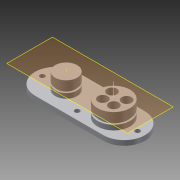
# Autodesk Inventor part: Connector
Saved by Autodesk Inventor 2014 SP2 (Build 180246200, 246)
## iProperties
Created: 2015-09-17
Part Number: Connector
Material: ABS Plastic
Document SubType Name: Modeling
Designer: Lukasz Szmit
Density: 1.06 g/cm^3
Appearance: Smooth - White
Author: Lukasz Szmit
Autodesk Inventor part; units mm, degrees
ref_plane "YZ Plane" through (0, 0, 0) normal (1, 0, 0) x (0, 1, 0)
ref_plane "XZ Plane" through (0, 0, 0) normal (0, 1, 0) x (-1, 0, 0)
sketch "Slot" plane through (0, 0, 0) normal (0, 0, 1) x (1, 0, 0)
  line L0 (-28, 17) -> (28, 17)
  line L1 (45, 0) -> (45, 0)
  line L2 (28, -17) -> (-28, -17)
  line L3 (-45, 0) -> (-45, 0)
  arc A0 (-28, 17) -> (-28, -17) centre (-28, 0) ccw
  arc A1 (28, -17) -> (28, 17) centre (28, 0) ccw
  point P0 (0, 0)
  point P1 (-45, 17)
  point P2 (45, 17)
  point P3 (-45, -17)
  dimension "d0" = 90
  dimension "d1" = 34
  dimension "d2" = 17
  dimension "d4" = 17
  dimension "d6" = 90
  dimension "d19" = 56
  dimension "d20" = 28
  constraints: 8 end point, 8 point on circle, 6 point on line, 4 tangent, 2 centre point, 2 perpendicular
  measures "d0" distance of point (-45, 17) point (45, 17)
  measures "d1" distance of point (-45, -17) point (-45, 17)
  measures "d2" distance from line of point (0, 0) L0
  measures "d4" radius of A0
  measures "d6" horizontal distance of point (45, 17) point (-45, -17)
  measures "d19" distance of A1.centre A0.centre
  measures "d20" distance of point (0, 0) A0.centre
sketch "Holes" plane through (0, 0, 0) normal (0, 0, 1) x (1, 0, 0)
  circle A0 centre (-39, 0) radius 2
  circle A1 centre (39, 0) radius 2
  circle A2 centre (0, -10.5) radius 2
  circle A3 centre (0, 10.5) radius 2
  point P0 (0, 0)
  point P1 (-3.3578, 23.5)
  dimension "d7" = 4
  dimension "d8" = 4
  dimension "d9" = 4
  dimension "d10" = 4
  dimension "d11" = 78
  dimension "d16" = 21
  dimension "d17" = 39
  constraints: 4 centre point
  measures "d7" diameter of A0
  measures "d8" diameter of A2
  measures "d9" diameter of A1
  measures "d10" diameter of A3
  measures "d11" distance of A1.centre A0.centre
  measures "d16" distance of A3.centre A2.centre
  measures "d17" horizontal distance of A1.centre A2.centre
extrude "Extrusion1" add sketch "Slot" against normal blind 4
hole "Hole1" at (0, 10.5, 0) at (39, 0, 0) at (0, -10.5, 0) at (-39, 0, 0) direction (0, 0, -1) diameter 4 end through all
ref_plane "Work Plane1" through (0, 0, 13) normal (0, 0, 1) x (1, 0, 0)
sketch "Socket Outline" plane through (0, 0, 13) normal (0, 0, 1) x (1, 0, 0)
  line L0 (-19.5, 12) -> (19.5, 12) construction
  line L1 (31.5, 0) -> (31.5, 0) construction
  line L2 (19.5, -12) -> (-19.5, -12) construction
  line L3 (-31.5, 0) -> (-31.5, 0) construction
  arc A0 (-19.5, 12) -> (-19.5, -12) centre (-19.5, 0) ccw construction
  arc A1 (19.5, -12) -> (19.5, 12) centre (19.5, 0) ccw construction
  point P0 (0, 0)
  point P1 (-31.5, 12)
  point P2 (31.5, 12)
  point P3 (-31.5, -12)
  dimension "d31" = 63
  dimension "d32" = 24
  dimension "d33" = 12
  dimension "d34" = 12
  dimension "d35" = 63
  dimension "d36" = 39
  dimension "d37" = 19.5
  constraints: 8 end point, 8 point on circle, 6 point on line, 4 tangent, 2 centre point, 2 perpendicular, 1 parallel
  measures "d31" distance of point (-31.5, 12) point (31.5, 12)
  measures "d32" distance of point (-31.5, -12) point (-31.5, 12)
  measures "d33" distance from line of point (0, 0) L0
  measures "d34" radius of A0
  measures "d35" horizontal distance of point (31.5, 12) point (-31.5, -12)
  measures "d36" distance of A1.centre A0.centre
  measures "d37" distance of point (0, 0) A0.centre
sketch "Small Socket" plane through (0, 0, 13) normal (0, 0, 1) x (1, 0, 0)
  circle A0 centre (-19.5, 0) radius 0.0027
  circle A1 centre (-19.5, 0) radius 9
  circle A2 centre (-39, 0) radius 2 projected
  point P0 (0, 0)
  dimension "d38" = 18
  dimension "d40" = 19.5
  dimension "d43" = 19.5
  constraints: 2 centre point, 1 coincident
  measures "d38" diameter of A1
  measures "d40" distance of A1.centre A2.centre
  measures "d43" distance of point (0, 0) A0.centre
sketch "Big Socket" plane through (0, 0, 13) normal (0, 0, 1) x (1, 0, 0)
  circle A0 centre (19.5, 0) radius 13.25
  circle A1 centre (39, 0) radius 2 projected
  point P0 (0, 0)
  dimension "d39" = 26.5
  dimension "d41" = 19.5
  dimension "d42" = 19.5
  constraints: 1 centre point
  measures "d39" diameter of A0
  measures "d41" distance of A1.centre A0.centre
  measures "d42" distance of point (0, 0) A0.centre
extrude "Extrusion2" add sketch "Small Socket" against normal blind 13 contours A1
extrude "Extrusion3" add sketch "Big Socket" against normal blind 13 contours A0
ref_plane "Work Plane3" through (-19.5, 0, 13) normal (1, 0, 0) x (0, 1, 0)
sketch "Sketch7" plane through (-19.5, 0, 13) normal (1, 0, 0) x (0, 1, 0)
  line L0 (-9, -13) -> (-9, 0) construction
  line L1 (-9, 0) -> (-0.0027, 0) construction
  line L2 (-0.0027, 0) -> (-0.0027, -13) construction
  line L3 (-0.0027, -13) -> (0.0027, -13) construction
  line L4 (0.0027, -13) -> (0.0027, 0) construction
  line L5 (0.0027, 0) -> (9, 0) construction
  line L6 (9, 0) -> (9, -13) construction
  line L7 (9, -13) -> (17, -13) construction
  line L8 (17, -13) -> (17, -17) construction
  line L9 (17, -17) -> (-17, -17) construction
  line L10 (-17, -17) -> (-17, -13) construction
  line L11 (-17, -13) -> (-9, -13) construction
  line L12 (9, -7.2) -> (7.5, -7.2)
  line L13 (7.5, -7.2) -> (7.5, -9)
  line L14 (7.5, -9) -> (9, -9)
  line L15 (9, -9) -> (9, -7.2)
  line L16 (0, 3.4) -> (0, -20.4) projected
  point P0 (0, -13)
  dimension "d53" = 1.5
  dimension "d54" = 1.8
  dimension "d55" = 4
  constraints: 8 end point, 1 perpendicular, 1 point on line
  measures "d53" distance of L12.start L12.end
  measures "d54" distance of L12.end L13.end
  measures "d55" distance between parallel lines of L7 L14
revolve "Revolution2" cut sketch "Sketch7" angle 360 about axis through (-19.5, 0, 13) along (0, 0, -1)
ref_plane "Work Plane4" through (19.5, 0, 13) normal (1, 0, 0) x (0, 1, 0)
sketch "Sketch8" plane through (19.5, 0, 13) normal (1, 0, 0) x (0, 1, 0)
  line L0 (-13.25, -13) -> (-13.25, 0) construction
  line L1 (-13.25, 0) -> (13.25, 0) construction
  line L2 (13.25, 0) -> (13.25, -13) construction
  line L3 (13.25, -13) -> (17, -13) construction
  line L4 (17, -13) -> (17, -17) construction
  line L5 (17, -17) -> (-17, -17) construction
  line L6 (-17, -17) -> (-17, -13) construction
  line L7 (-17, -13) -> (-13.25, -13) construction
  line L8 (-13.25, -7.2) -> (-11.75, -7.2)
  line L9 (-11.75, -7.2) -> (-11.75, -9)
  line L10 (-11.75, -9) -> (-13.25, -9)
  line L11 (-13.25, -9) -> (-13.25, -7.2)
  line L12 (0, 3.4) -> (0, -20.4) projected
  point P0 (0, -13)
  dimension "d57" = 1.5
  dimension "d58" = 1.8
  dimension "d59" = 4
  constraints: 8 end point, 2 perpendicular, 1 parallel, 1 point on line
  measures "d57" distance of L8.start L8.end
  measures "d58" distance of L8.end L9.end
  measures "d59" distance from line of L0.start L10
revolve "Revolution3" cut sketch "Sketch8" angle 360 about axis through (19.5, 0, 13) along (0, 0, -1)
ref_plane "Work Plane5" through (0, 0, 13) normal (0, 0, 1) x (1, 0, 0)
sketch "Sketch9" plane through (19.5, 0, 13) normal (0, 0, 1) x (1, 0, 0)
  circle A0 centre (0, 0) radius 13.25 construction
  circle A1 centre (-6, 4.5) radius 4
  circle A2 centre (6, 4.5) radius 4
  circle A3 centre (-4.5, -4.5) radius 4
  circle A4 centre (4.5, -4.5) radius 4
  point P0 (-19.5, 0)
  dimension "d62" = 8
  dimension "d63" = 6
  dimension "d64" = 4.5
  dimension "d65" = 4.5
  dimension "d66" = 4.5
  dimension "d67" = 4.5
  dimension "d68" = 6
  dimension "d69" = 8
  dimension "d70" = 8
  dimension "d71" = 8
  dimension "d72" = 4.5
  dimension "d73" = 4.5
  constraints: 4 centre point
  measures "d62" diameter of A1
  measures "d63" horizontal distance of A0.centre A1.centre
  measures "d64" vertical distance of A0.centre A1.centre
  measures "d65" horizontal distance of A3.centre A0.centre
  measures "d66" vertical distance of A0.centre A2.centre
  measures "d67" horizontal distance of A0.centre A4.centre
  measures "d68" horizontal distance of A0.centre A2.centre
  measures "d69" diameter of A2
  measures "d70" diameter of A3
  measures "d71" diameter of A4
  measures "d72" horizontal distance of A0.centre A3.centre
  measures "d73" horizontal distance of A4.centre A0.centre
hole "Hole2" at (24, -4.5, 13) at (15, -4.5, 13) at (13.5, 4.5, 13) at (25.5, 4.5, 13) direction (0, 0, -1) diameter 8 depth 13
sketch "Sketch10" plane through (19.5, 0, 13) normal (0, 0, 1) x (1, 0, 0)
  circle A0 centre (0, 0) radius 13.25 projected
  circle A1 centre (0, 0) radius 0.375
  point P0 (-19.5, 0)
  dimension "d88" = 0.75
  constraints: 1 centre point, 1 coincident
  measures "d88" diameter of A1
hole "Hole3" at (19.5, 0, 13) direction (0, 0, -1) diameter 0.75 end through all
equation "\"d2\" = 0.5 * d1"
equation "\"d4\" = 0.5 * d1"
equation "\"d6\" = d0"
equation "\"d19\" = d0 - 2 * d4"
equation "\"d20\" = 0.5 * d19"
equation "\"d8\" = d7"
equation "\"d9\" = d7"
equation "\"d10\" = d7"
equation "\"d33\" = 0.5 * d32"
equation "\"d34\" = 0.5 * d32"
equation "\"d35\" = d31"
equation "\"d36\" = d31 - 2 * d34"
equation "\"d37\" = 0.5 * d36"
equation "\"d40\" = d41"
equation "\"d43\" = d41"
equation "\"d42\" = d41"
equation "\"d65\" = d64"
equation "\"d66\" = d64"
equation "\"d67\" = d64"
equation "\"d68\" = d63"
equation "\"d69\" = d62"
equation "\"d70\" = d62"
equation "\"d71\" = d62"
equation "\"d73\" = d72"
body "Solid1"
